Autodesk Inventor part; units mm, degrees
(part 2 of 4)
sketch "Sketch5" plane through (0, 0, 0) normal (-1, 0, 0) x (0, 0, 1)
  line L0 (0, 0) -> (304.8, 0) projected
  line L1 (0, 0) -> (0, -25.4) projected
  line L2 (304.8, -25.4) -> (0, -25.4) projected
  line L3 (304.8, 0) -> (304.8, -25.4) projected
  line L4 (24.765, -3.175) -> (24.765, -22.225)
  line L5 (24.765, -22.225) -> (26.035, -22.225)
  line L6 (26.035, -22.225) -> (26.035, -3.175)
  line L7 (26.035, -3.175) -> (24.765, -3.175)
  line L8 (6.0325, -6.35) -> (18.7325, -6.35) construction
  line L9 (18.7325, -6.35) -> (18.7325, -19.05) construction
  line L10 (18.7325, -19.05) -> (6.0325, -19.05) construction
  line L11 (6.0325, -19.05) -> (6.0325, -6.35) construction
  line L12 (50.165, -3.175) -> (50.165, -22.225)
  line L13 (51.435, -3.175) -> (50.165, -3.175)
  line L14 (50.165, -22.225) -> (51.435, -22.225)
  line L15 (51.435, -22.225) -> (51.435, -3.175)
  line L16 (75.565, -3.175) -> (75.565, -22.225)
  line L17 (76.835, -3.175) -> (75.565, -3.175)
  line L18 (75.565, -22.225) -> (76.835, -22.225)
  line L19 (76.835, -22.225) -> (76.835, -3.175)
  line L20 (100.965, -3.175) -> (100.965, -22.225)
  line L21 (102.235, -3.175) -> (100.965, -3.175)
  line L22 (100.965, -22.225) -> (102.235, -22.225)
  line L23 (102.235, -22.225) -> (102.235, -3.175)
  line L24 (126.365, -3.175) -> (126.365, -22.225)
  line L25 (127.635, -3.175) -> (126.365, -3.175)
  line L26 (126.365, -22.225) -> (127.635, -22.225)
  line L27 (127.635, -22.225) -> (127.635, -3.175)
  line L28 (151.765, -3.175) -> (151.765, -22.225)
  line L29 (153.035, -3.175) -> (151.765, -3.175)
  line L30 (151.765, -22.225) -> (153.035, -22.225)
  line L31 (153.035, -22.225) -> (153.035, -3.175)
  line L32 (177.165, -3.175) -> (177.165, -22.225)
  line L33 (178.435, -3.175) -> (177.165, -3.175)
  line L34 (177.165, -22.225) -> (178.435, -22.225)
  line L35 (178.435, -22.225) -> (178.435, -3.175)
  line L36 (202.565, -3.175) -> (202.565, -22.225)
  line L37 (203.835, -3.175) -> (202.565, -3.175)
  line L38 (202.565, -22.225) -> (203.835, -22.225)
  line L39 (203.835, -22.225) -> (203.835, -3.175)
  line L40 (227.965, -3.175) -> (227.965, -22.225)
  line L41 (229.235, -3.175) -> (227.965, -3.175)
  line L42 (227.965, -22.225) -> (229.235, -22.225)
  line L43 (229.235, -22.225) -> (229.235, -3.175)
  line L44 (253.365, -3.175) -> (253.365, -22.225)
  line L45 (254.635, -3.175) -> (253.365, -3.175)
  line L46 (253.365, -22.225) -> (254.635, -22.225)
  line L47 (254.635, -22.225) -> (254.635, -3.175)
  line L48 (278.765, -3.175) -> (278.765, -22.225)
  line L49 (280.035, -3.175) -> (278.765, -3.175)
  line L50 (278.765, -22.225) -> (280.035, -22.225)
  line L51 (280.035, -22.225) -> (280.035, -3.175)
  line L52 (31.4325, -6.35) -> (44.1325, -6.35) construction
  line L53 (44.1325, -6.35) -> (44.1325, -19.05) construction
  line L54 (44.1325, -19.05) -> (31.4325, -19.05) construction
  line L55 (31.4325, -19.05) -> (31.4325, -6.35) construction
  line L56 (56.8325, -6.35) -> (69.5325, -6.35) construction
  line L57 (69.5325, -6.35) -> (69.5325, -19.05) construction
  line L58 (69.5325, -19.05) -> (56.8325, -19.05) construction
  line L59 (56.8325, -19.05) -> (56.8325, -6.35) construction
  line L60 (82.2325, -6.35) -> (94.9325, -6.35) construction
  line L61 (94.9325, -6.35) -> (94.9325, -19.05) construction
  line L62 (94.9325, -19.05) -> (82.2325, -19.05) construction
  line L63 (82.2325, -19.05) -> (82.2325, -6.35) construction
  line L64 (107.6325, -6.35) -> (120.3325, -6.35) construction
  line L65 (120.3325, -6.35) -> (120.3325, -19.05) construction
  line L66 (120.3325, -19.05) -> (107.6325, -19.05) construction
  line L67 (107.6325, -19.05) -> (107.6325, -6.35) construction
  line L68 (133.0325, -6.35) -> (145.7325, -6.35) construction
  line L69 (145.7325, -6.35) -> (145.7325, -19.05) construction
  line L70 (145.7325, -19.05) -> (133.0325, -19.05) construction
  line L71 (133.0325, -19.05) -> (133.0325, -6.35) construction
  line L72 (158.4325, -6.35) -> (171.1325, -6.35) construction
  line L73 (171.1325, -6.35) -> (171.1325, -19.05) construction
  line L74 (171.1325, -19.05) -> (158.4325, -19.05) construction
  line L75 (158.4325, -19.05) -> (158.4325, -6.35) construction
  line L76 (183.8325, -6.35) -> (196.5325, -6.35) construction
  line L77 (196.5325, -6.35) -> (196.5325, -19.05) construction
  line L78 (196.5325, -19.05) -> (183.8325, -19.05) construction
  line L79 (183.8325, -19.05) -> (183.8325, -6.35) construction
  line L80 (209.2325, -6.35) -> (221.9325, -6.35) construction
  line L81 (221.9325, -6.35) -> (221.9325, -19.05) construction
  line L82 (221.9325, -19.05) -> (209.2325, -19.05) construction
  line L83 (209.2325, -19.05) -> (209.2325, -6.35) construction
  line L84 (234.6325, -6.35) -> (247.3325, -6.35) construction
  line L85 (247.3325, -6.35) -> (247.3325, -19.05) construction
  line L86 (247.3325, -19.05) -> (234.6325, -19.05) construction
  line L87 (234.6325, -19.05) -> (234.6325, -6.35) construction
  line L88 (260.0325, -6.35) -> (272.7325, -6.35) construction
  line L89 (272.7325, -6.35) -> (272.7325, -19.05) construction
  line L90 (272.7325, -19.05) -> (260.0325, -19.05) construction
  line L91 (260.0325, -19.05) -> (260.0325, -6.35) construction
  line L92 (285.4325, -6.35) -> (298.1325, -6.35) construction
  line L93 (298.1325, -6.35) -> (298.1325, -19.05) construction
  line L94 (298.1325, -19.05) -> (285.4325, -19.05) construction
  line L95 (285.4325, -19.05) -> (285.4325, -6.35) construction
  line L96 (29.3758, -17.272) -> (32.4584, -8.128)
  line L97 (32.4584, -8.128) -> (33.9552, -8.128)
  line L98 (33.9552, -8.128) -> (37.0378, -17.272)
  line L99 (37.0378, -17.272) -> (35.7559, -17.272)
  line L100 (35.7559, -17.272) -> (34.9259, -14.7155)
  line L101 (34.9259, -14.7155) -> (31.4358, -14.7155)
  line L102 (31.4358, -14.7155) -> (30.6059, -17.272)
  line L103 (30.6059, -17.272) -> (29.3758, -17.272)
  line L104 (34.5925, -13.6781) -> (33.1772, -9.3729)
  line L105 (33.1772, -9.3729) -> (31.7692, -13.6781)
  line L106 (31.7692, -13.6781) -> (34.5925, -13.6781)
  line L107 (45.2629, -11.5514) -> (43.4623, -11.5514)
  line L108 (43.4623, -11.5514) -> (42.9065, -13.856)
  line L109 (42.9065, -13.856) -> (44.5442, -13.856)
  line L110 (44.5442, -13.856) -> (44.5442, -14.6859)
  line L111 (44.5442, -14.6859) -> (42.6917, -14.6859)
  line L112 (42.6917, -14.6859) -> (42.047, -17.272)
  line L113 (42.047, -17.272) -> (41.2541, -17.272)
  line L114 (41.2541, -17.272) -> (41.8988, -14.6859)
  line L115 (41.8988, -14.6859) -> (40.2241, -14.6859)
  line L116 (40.2241, -14.6859) -> (39.5794, -17.272)
  line L117 (39.5794, -17.272) -> (38.7866, -17.272)
  line L118 (38.7866, -17.272) -> (39.4312, -14.6859)
  line L119 (39.4312, -14.6859) -> (37.8455, -14.6859)
  line L120 (37.8455, -14.6859) -> (37.8455, -13.856)
  line L121 (37.8455, -13.856) -> (39.6461, -13.856)
  line L122 (39.6461, -13.856) -> (40.2019, -11.5514)
  line L123 (40.2019, -11.5514) -> (38.5643, -11.5514)
  line L124 (38.5643, -11.5514) -> (38.5643, -10.7215)
  line L125 (38.5643, -10.7215) -> (40.4168, -10.7215)
  line L126 (40.4168, -10.7215) -> (41.0614, -8.128)
  line L127 (41.0614, -8.128) -> (41.8543, -8.128)
  line L128 (41.8543, -8.128) -> (41.2096, -10.7215)
  line L129 (41.2096, -10.7215) -> (42.8843, -10.7215)
  line L130 (42.8843, -10.7215) -> (43.529, -8.128)
  line L131 (43.529, -8.128) -> (44.3219, -8.128)
  line L132 (44.3219, -8.128) -> (43.6772, -10.7215)
  line L133 (43.6772, -10.7215) -> (45.2629, -10.7215)
  line L134 (45.2629, -10.7215) -> (45.2629, -11.5514)
  line L135 (42.6917, -11.5366) -> (40.9948, -11.5366)
  line L136 (40.9948, -11.5366) -> (40.4242, -13.8708)
  line L137 (40.4242, -13.8708) -> (42.1211, -13.8708)
  line L138 (42.1211, -13.8708) -> (42.6917, -11.5366)
  spline S0 degree 2 poles (15.8059, -14.4636) (15.8059, -15.1453) (15.2872, -16.1901) (14.8575, -16.531) knots 0 0 0 1 2 2 2
  spline S1 degree 2 poles (14.8575, -16.531) (14.3388, -16.9311) (13.1606, -17.272) (12.2269, -17.272) knots 0 0 0 1 2 2 2
  line L139 (12.2269, -17.272) -> (9.6037, -17.272)
  line L140 (9.6037, -17.272) -> (9.6037, -8.128)
  line L141 (9.6037, -8.128) -> (12.0268, -8.128)
  spline S2 degree 2 poles (12.0268, -8.128) (13.0049, -8.128) (13.9831, -8.254) (14.4277, -8.4985) knots 0 0 0 1 2 2 2
  spline S3 degree 2 poles (14.4277, -8.4985) (14.9241, -8.7579) (15.3762, -9.61) (15.3762, -10.188) knots 0 0 0 1 2 2 2
  spline S4 degree 2 poles (15.3762, -10.188) (15.3762, -10.8327) (14.6944, -11.8553) (14.0942, -12.1442) knots 0 0 0 1 2 2 2
  line L142 (14.0942, -12.1442) -> (14.0942, -12.1887)
  spline S5 degree 2 poles (14.0942, -12.1887) (14.9093, -12.411) (15.8059, -13.5892) (15.8059, -14.4636) knots 0 0 0 1 2 2 2
  spline S6 degree 2 poles (14.5388, -14.5155) (14.5388, -13.9968) (14.2424, -13.3299) (13.7978, -13.0927) knots 0 0 0 1 2 2 2
  spline S7 degree 2 poles (13.7978, -13.0927) (13.5088, -12.9445) (12.8271, -12.8556) (12.1972, -12.8556) knots 0 0 0 1 2 2 2
  line L143 (12.1972, -12.8556) -> (10.819, -12.8556)
  line L144 (10.819, -12.8556) -> (10.819, -16.2346)
  line L145 (10.819, -16.2346) -> (11.8045, -16.2346)
  spline S8 degree 2 poles (11.8045, -16.2346) (12.6048, -16.2346) (13.5236, -16.0864) (13.8793, -15.8493) knots 0 0 0 1 2 2 2
  spline S9 degree 2 poles (13.8793, -15.8493) (14.2202, -15.6047) (14.5388, -14.9971) (14.5388, -14.5155) knots 0 0 0 1 2 2 2
  spline S10 degree 2 poles (14.109, -10.3584) (14.109, -10.0324) (13.8867, -9.5433) (13.6422, -9.4025) knots 0 0 0 1 2 2 2
  spline S11 degree 2 poles (13.6422, -9.4025) (13.3458, -9.2395) (12.627, -9.1654) (11.9824, -9.1654) knots 0 0 0 1 2 2 2
  line L146 (11.9824, -9.1654) -> (10.819, -9.1654)
  line L147 (10.819, -9.1654) -> (10.819, -11.8404)
  line L148 (10.819, -11.8404) -> (12.1972, -11.8404)
  spline S12 degree 2 poles (12.1972, -11.8404) (12.7678, -11.8404) (13.3088, -11.7219) (13.5977, -11.5366) knots 0 0 0 1 2 2 2
  spline S13 degree 2 poles (13.5977, -11.5366) (13.8793, -11.3588) (14.109, -10.7882) (14.109, -10.3584) knots 0 0 0 1 2 2 2
  line L149 (59.2922, -17.272) -> (62.3748, -8.128)
  line L150 (62.3748, -8.128) -> (63.8716, -8.128)
  line L151 (63.8716, -8.128) -> (66.9542, -17.272)
  line L152 (66.9542, -17.272) -> (65.6723, -17.272)
  line L153 (65.6723, -17.272) -> (64.8424, -14.7155)
  line L154 (64.8424, -14.7155) -> (61.3522, -14.7155)
  line L155 (61.3522, -14.7155) -> (60.5223, -17.272)
  line L156 (60.5223, -17.272) -> (59.2922, -17.272)
  line L157 (64.5089, -13.6781) -> (63.0936, -9.3729)
  line L158 (63.0936, -9.3729) -> (61.6857, -13.6781)
  line L159 (61.6857, -13.6781) -> (64.5089, -13.6781)
  spline S14 degree 2 poles (84.5663, -17.4424) (83.5955, -17.4424) (81.9876, -16.8496) (81.4096, -16.2494) knots 0 0 0 1 2 2 2
  spline S15 degree 2 poles (81.4096, -16.2494) (80.8316, -15.6418) (80.2166, -13.8486) (80.2166, -12.6852) knots 0 0 0 1 2 2 2
  spline S16 degree 2 poles (80.2166, -12.6852) (80.2166, -11.5811) (80.839, -9.8323) (81.417, -9.2099) knots 0 0 0 1 2 2 2
  spline S17 degree 2 poles (81.417, -9.2099) (81.9727, -8.6097) (83.6029, -7.9576) (84.5737, -7.9576) knots 0 0 0 1 2 2 2
  spline S18 degree 2 poles (84.5737, -7.9576) (85.0405, -7.9576) (85.8852, -8.0909) (86.2706, -8.2095) knots 0 0 0 1 2 2 2
  spline S19 degree 2 poles (86.2706, -8.2095) (86.5818, -8.2984) (87.3376, -8.6245) (87.5673, -8.743) knots 0 0 0 1 2 2 2
  line L160 (87.5673, -8.743) -> (87.5673, -10.2102)
  line L161 (87.5673, -10.2102) -> (87.4636, -10.2102)
  spline S20 degree 2 poles (87.4636, -10.2102) (87.2339, -10.0102) (86.7522, -9.6471) (86.3076, -9.4396) knots 0 0 0 1 2 2 2
  spline S21 degree 2 poles (86.3076, -9.4396) (85.9371, -9.2543) (84.9812, -9.0098) (84.4329, -9.0098) knots 0 0 0 1 2 2 2
  spline S22 degree 2 poles (84.4329, -9.0098) (83.1139, -9.0098) (81.4837, -10.9957) (81.4837, -12.6481) knots 0 0 0 1 2 2 2
  spline S23 degree 2 poles (81.4837, -12.6481) (81.4837, -13.567) (81.9135, -14.9452) (82.321, -15.4195) knots 0 0 0 1 2 2 2
  spline S24 degree 2 poles (82.321, -15.4195) (82.7137, -15.8937) (83.8252, -16.3902) (84.5218, -16.3902) knots 0 0 0 1 2 2 2
  spline S25 degree 2 poles (84.5218, -16.3902) (85.0331, -16.3902) (86.0557, -16.242) (86.4039, -16.0938) knots 0 0 0 1 2 2 2
  line L162 (86.4039, -16.0938) -> (86.4039, -13.73)
  line L163 (86.4039, -13.73) -> (84.2847, -13.73)
  line L164 (84.2847, -13.73) -> (84.2847, -12.6629)
  line L165 (84.2847, -12.6629) -> (87.6044, -12.6629)
  line L166 (87.6044, -12.6629) -> (87.6044, -16.657)
  spline S26 degree 2 poles (87.6044, -16.657) (87.3747, -16.7607) (86.5892, -17.0793) (86.2557, -17.1757) knots 0 0 0 1 2 2 2
  spline S27 degree 2 poles (86.2557, -17.1757) (85.8037, -17.3091) (85.0775, -17.4424) (84.5663, -17.4424) knots 0 0 0 1 2 2 2
  line L167 (96.489, -11.544) -> (94.6884, -11.544)
  line L168 (94.6884, -11.544) -> (94.1326, -13.8486)
  line L169 (94.1326, -13.8486) -> (95.7702, -13.8486)
  line L170 (95.7702, -13.8486) -> (95.7702, -14.6785)
  line L171 (95.7702, -14.6785) -> (93.9177, -14.6785)
  line L172 (93.9177, -14.6785) -> (93.2731, -17.2646)
  line L173 (93.2731, -17.2646) -> (92.4802, -17.2646)
  line L174 (92.4802, -17.2646) -> (93.1249, -14.6785)
  line L175 (93.1249, -14.6785) -> (91.4502, -14.6785)
  line L176 (91.4502, -14.6785) -> (90.8055, -17.2646)
  line L177 (90.8055, -17.2646) -> (90.0126, -17.2646)
  line L178 (90.0126, -17.2646) -> (90.6573, -14.6785)
  line L179 (90.6573, -14.6785) -> (89.0716, -14.6785)
  line L180 (89.0716, -14.6785) -> (89.0716, -13.8486)
  line L181 (89.0716, -13.8486) -> (90.8722, -13.8486)
  line L182 (90.8722, -13.8486) -> (91.428, -11.544)
  line L183 (91.428, -11.544) -> (89.7903, -11.544)
  line L184 (89.7903, -11.544) -> (89.7903, -10.7141)
  line L185 (89.7903, -10.7141) -> (91.6428, -10.7141)
  line L186 (91.6428, -10.7141) -> (92.2875, -8.1206)
  line L187 (92.2875, -8.1206) -> (93.0804, -8.1206)
  line L188 (93.0804, -8.1206) -> (92.4357, -10.7141)
  line L189 (92.4357, -10.7141) -> (94.1104, -10.7141)
  line L190 (94.1104, -10.7141) -> (94.7551, -8.1206)
  line L191 (94.7551, -8.1206) -> (95.5479, -8.1206)
  line L192 (95.5479, -8.1206) -> (94.9033, -10.7141)
  line L193 (94.9033, -10.7141) -> (96.489, -10.7141)
  line L194 (96.489, -10.7141) -> (96.489, -11.544)
  line L195 (93.9177, -11.5292) -> (92.2208, -11.5292)
  line L196 (92.2208, -11.5292) -> (91.6503, -13.8634)
  line L197 (91.6503, -13.8634) -> (93.3472, -13.8634)
  line L198 (93.3472, -13.8634) -> (93.9177, -11.5292)
  spline S28 degree 2 poles (114.542, -17.4424) (113.5712, -17.4424) (111.9633, -16.8496) (111.3853, -16.2494) knots 0 0 0 1 2 2 2
  spline S29 degree 2 poles (111.3853, -16.2494) (110.8073, -15.6418) (110.1923, -13.8486) (110.1923, -12.6852) knots 0 0 0 1 2 2 2
  spline S30 degree 2 poles (110.1923, -12.6852) (110.1923, -11.5811) (110.8147, -9.8323) (111.3927, -9.2099) knots 0 0 0 1 2 2 2
  spline S31 degree 2 poles (111.3927, -9.2099) (111.9484, -8.6097) (113.5787, -7.9576) (114.5494, -7.9576) knots 0 0 0 1 2 2 2
  spline S32 degree 2 poles (114.5494, -7.9576) (115.0162, -7.9576) (115.8609, -8.0909) (116.2463, -8.2095) knots 0 0 0 1 2 2 2
  spline S33 degree 2 poles (116.2463, -8.2095) (116.5575, -8.2984) (117.3133, -8.6245) (117.543, -8.743) knots 0 0 0 1 2 2 2
  line L199 (117.543, -8.743) -> (117.543, -10.2102)
  line L200 (117.543, -10.2102) -> (117.4393, -10.2102)
  spline S34 degree 2 poles (117.4393, -10.2102) (117.2096, -10.0102) (116.7279, -9.6471) (116.2833, -9.4396) knots 0 0 0 1 2 2 2
  spline S35 degree 2 poles (116.2833, -9.4396) (115.9128, -9.2543) (114.9569, -9.0098) (114.4086, -9.0098) knots 0 0 0 1 2 2 2
  spline S36 degree 2 poles (114.4086, -9.0098) (113.0896, -9.0098) (111.4594, -10.9957) (111.4594, -12.6481) knots 0 0 0 1 2 2 2
  spline S37 degree 2 poles (111.4594, -12.6481) (111.4594, -13.567) (111.8892, -14.9452) (112.2967, -15.4195) knots 0 0 0 1 2 2 2
  spline S38 degree 2 poles (112.2967, -15.4195) (112.6894, -15.8937) (113.801, -16.3902) (114.4975, -16.3902) knots 0 0 0 1 2 2 2
  spline S39 degree 2 poles (114.4975, -16.3902) (115.0088, -16.3902) (116.0314, -16.242) (116.3796, -16.0938) knots 0 0 0 1 2 2 2
  line L201 (116.3796, -16.0938) -> (116.3796, -13.73)
  line L202 (116.3796, -13.73) -> (114.2604, -13.73)
  line L203 (114.2604, -13.73) -> (114.2604, -12.6629)
  line L204 (114.2604, -12.6629) -> (117.5801, -12.6629)
  line L205 (117.5801, -12.6629) -> (117.5801, -16.657)
  spline S40 degree 2 poles (117.5801, -16.657) (117.3504, -16.7607) (116.5649, -17.0793) (116.2314, -17.1757) knots 0 0 0 1 2 2 2
  spline S41 degree 2 poles (116.2314, -17.1757) (115.7794, -17.3091) (115.0533, -17.4424) (114.542, -17.4424) knots 0 0 0 1 2 2 2
  line L206 (137.9227, -9.2099) -> (133.6694, -9.2099)
  line L207 (133.6694, -9.2099) -> (133.6694, -11.7886)
  line L208 (133.6694, -11.7886) -> (137.7449, -11.7886)
  line L209 (137.7449, -11.7886) -> (137.7449, -12.8704)
  line L210 (137.7449, -12.8704) -> (133.6694, -12.8704)
  line L211 (133.6694, -12.8704) -> (133.6694, -17.272)
  line L212 (133.6694, -17.272) -> (132.4541, -17.272)
  line L213 (132.4541, -17.272) -> (132.4541, -8.128)
  line L214 (132.4541, -8.128) -> (137.9227, -8.128)
  line L215 (137.9227, -8.128) -> (137.9227, -9.2099)
  line L216 (146.3702, -11.5514) -> (144.5695, -11.5514)
  line L217 (144.5695, -11.5514) -> (144.0138, -13.856)
  line L218 (144.0138, -13.856) -> (145.6514, -13.856)
  line L219 (145.6514, -13.856) -> (145.6514, -14.6859)
  line L220 (145.6514, -14.6859) -> (143.7989, -14.6859)
  line L221 (143.7989, -14.6859) -> (143.1542, -17.272)
  line L222 (143.1542, -17.272) -> (142.3613, -17.272)
  line L223 (142.3613, -17.272) -> (143.006, -14.6859)
  line L224 (143.006, -14.6859) -> (141.3313, -14.6859)
  line L225 (141.3313, -14.6859) -> (140.6867, -17.272)
  line L226 (140.6867, -17.272) -> (139.8938, -17.272)
  line L227 (139.8938, -17.272) -> (140.5385, -14.6859)
  line L228 (140.5385, -14.6859) -> (138.9527, -14.6859)
  line L229 (138.9527, -14.6859) -> (138.9527, -13.856)
  line L230 (138.9527, -13.856) -> (140.7534, -13.856)
  line L231 (140.7534, -13.856) -> (141.3091, -11.5514)
  line L232 (141.3091, -11.5514) -> (139.6715, -11.5514)
  line L233 (139.6715, -11.5514) -> (139.6715, -10.7215)
  line L234 (139.6715, -10.7215) -> (141.524, -10.7215)
  line L235 (141.524, -10.7215) -> (142.1687, -8.128)
  line L236 (142.1687, -8.128) -> (142.9616, -8.128)
  line L237 (142.9616, -8.128) -> (142.3169, -10.7215)
  line L238 (142.3169, -10.7215) -> (143.9915, -10.7215)
  line L239 (143.9915, -10.7215) -> (144.6362, -8.128)
  line L240 (144.6362, -8.128) -> (145.4291, -8.128)
  line L241 (145.4291, -8.128) -> (144.7844, -10.7215)
  line L242 (144.7844, -10.7215) -> (146.3702, -10.7215)
  line L243 (146.3702, -10.7215) -> (146.3702, -11.5514)
  line L244 (143.7989, -11.5366) -> (142.102, -11.5366)
  line L245 (142.102, -11.5366) -> (141.5314, -13.8708)
  line L246 (141.5314, -13.8708) -> (143.2283, -13.8708)
  line L247 (143.2283, -13.8708) -> (143.7989, -11.5366)
  line L248 (167.8984, -9.2099) -> (163.6451, -9.2099)
  line L249 (163.6451, -9.2099) -> (163.6451, -11.7886)
  line L250 (163.6451, -11.7886) -> (167.7206, -11.7886)
  line L251 (167.7206, -11.7886) -> (167.7206, -12.8704)
  line L252 (167.7206, -12.8704) -> (163.6451, -12.8704)
  line L253 (163.6451, -12.8704) -> (163.6451, -17.272)
  line L254 (163.6451, -17.272) -> (162.4298, -17.272)
  line L255 (162.4298, -17.272) -> (162.4298, -8.128)
  line L256 (162.4298, -8.128) -> (167.8984, -8.128)
  line L257 (167.8984, -8.128) -> (167.8984, -9.2099)
  line L258 (187.5816, -17.272) -> (187.5816, -8.128)
  line L259 (187.5816, -8.128) -> (193.3021, -8.128)
  line L260 (193.3021, -8.128) -> (193.3021, -9.2099)
  line L261 (193.3021, -9.2099) -> (188.7968, -9.2099)
  line L262 (188.7968, -9.2099) -> (188.7968, -11.7145)
  line L263 (188.7968, -11.7145) -> (192.9983, -11.7145)
  line L264 (192.9983, -11.7145) -> (192.9983, -12.7963)
  line L265 (192.9983, -12.7963) -> (188.7968, -12.7963)
  line L266 (188.7968, -12.7963) -> (188.7968, -16.1901)
  line L267 (188.7968, -16.1901) -> (193.3021, -16.1901)
  line L268 (193.3021, -16.1901) -> (193.3021, -17.272)
  line L269 (193.3021, -17.272) -> (187.5816, -17.272)
  spline S42 degree 2 poles (214.8785, -12.7074) (214.8785, -13.9597) (213.8634, -15.9752) (213.0112, -16.5384) knots 0 0 0 1 2 2 2
  spline S43 degree 2 poles (213.0112, -16.5384) (212.3147, -16.9756) (210.8845, -17.272) (209.773, -17.272) knots 0 0 0 1 2 2 2
  line L270 (209.773, -17.272) -> (207.6686, -17.272)
  line L271 (207.6686, -17.272) -> (207.6686, -8.128)
  line L272 (207.6686, -8.128) -> (209.7508, -8.128)
  spline S44 degree 2 poles (209.7508, -8.128) (211.0401, -8.128) (212.5073, -8.5133) (213.026, -8.8542) knots 0 0 0 1 2 2 2
  spline S45 degree 2 poles (213.026, -8.8542) (213.9078, -9.4396) (214.8785, -11.3736) (214.8785, -12.7074) knots 0 0 0 1 2 2 2
  spline S46 degree 2 poles (213.6114, -12.6926) (213.6114, -11.6404) (212.9149, -10.1509) (212.2257, -9.7286) knots 0 0 0 1 2 2 2
  spline S47 degree 2 poles (212.2257, -9.7286) (211.7367, -9.4396) (210.6326, -9.1802) (209.8101, -9.1802) knots 0 0 0 1 2 2 2
  line L273 (209.8101, -9.1802) -> (208.8838, -9.1802)
  line L274 (208.8838, -9.1802) -> (208.8838, -16.2198)
  line L275 (208.8838, -16.2198) -> (209.8101, -16.2198)
  spline S48 degree 2 poles (209.8101, -16.2198) (210.6178, -16.2198) (211.8404, -15.9604) (212.3369, -15.6121) knots 0 0 0 1 2 2 2
  spline S49 degree 2 poles (212.3369, -15.6121) (212.9742, -15.1824) (213.6114, -13.7596) (213.6114, -12.6926) knots 0 0 0 1 2 2 2
  line L276 (223.5557, -11.5514) -> (221.7551, -11.5514)
  line L277 (221.7551, -11.5514) -> (221.1993, -13.856)
  line L278 (221.1993, -13.856) -> (222.8369, -13.856)
  line L279 (222.8369, -13.856) -> (222.8369, -14.6859)
  line L280 (222.8369, -14.6859) -> (220.9844, -14.6859)
  line L281 (220.9844, -14.6859) -> (220.3397, -17.272)
  line L282 (220.3397, -17.272) -> (219.5469, -17.272)
  line L283 (219.5469, -17.272) -> (220.1915, -14.6859)
  line L284 (220.1915, -14.6859) -> (218.5169, -14.6859)
  line L285 (218.5169, -14.6859) -> (217.8722, -17.272)
  line L286 (217.8722, -17.272) -> (217.0793, -17.272)
  line L287 (217.0793, -17.272) -> (217.724, -14.6859)
  line L288 (217.724, -14.6859) -> (216.1383, -14.6859)
  line L289 (216.1383, -14.6859) -> (216.1383, -13.856)
  line L290 (216.1383, -13.856) -> (217.9389, -13.856)
  line L291 (217.9389, -13.856) -> (218.4946, -11.5514)
  line L292 (218.4946, -11.5514) -> (216.857, -11.5514)
  line L293 (216.857, -11.5514) -> (216.857, -10.7215)
  line L294 (216.857, -10.7215) -> (218.7095, -10.7215)
  line L295 (218.7095, -10.7215) -> (219.3542, -8.128)
  line L296 (219.3542, -8.128) -> (220.1471, -8.128)
  line L297 (220.1471, -8.128) -> (219.5024, -10.7215)
  line L298 (219.5024, -10.7215) -> (221.1771, -10.7215)
  line L299 (221.1771, -10.7215) -> (221.8218, -8.128)
  line L300 (221.8218, -8.128) -> (222.6146, -8.128)
  line L301 (222.6146, -8.128) -> (221.97, -10.7215)
  line L302 (221.97, -10.7215) -> (223.5557, -10.7215)
  line L303 (223.5557, -10.7215) -> (223.5557, -11.5514)
  line L304 (220.9844, -11.5366) -> (219.2875, -11.5366)
  line L305 (219.2875, -11.5366) -> (218.7169, -13.8708)
  line L306 (218.7169, -13.8708) -> (220.4138, -13.8708)
  line L307 (220.4138, -13.8708) -> (220.9844, -11.5366)
  spline S50 degree 2 poles (244.8542, -12.7074) (244.8542, -13.9597) (243.8391, -15.9752) (242.9869, -16.5384) knots 0 0 0 1 2 2 2
  spline S51 degree 2 poles (242.9869, -16.5384) (242.2904, -16.9756) (240.8602, -17.272) (239.7487, -17.272) knots 0 0 0 1 2 2 2
  line L308 (239.7487, -17.272) -> (237.6443, -17.272)
  line L309 (237.6443, -17.272) -> (237.6443, -8.128)
  line L310 (237.6443, -8.128) -> (239.7265, -8.128)
  spline S52 degree 2 poles (239.7265, -8.128) (241.0158, -8.128) (242.483, -8.5133) (243.0017, -8.8542) knots 0 0 0 1 2 2 2
  spline S53 degree 2 poles (243.0017, -8.8542) (243.8835, -9.4396) (244.8542, -11.3736) (244.8542, -12.7074) knots 0 0 0 1 2 2 2
  spline S54 degree 2 poles (243.5871, -12.6926) (243.5871, -11.6404) (242.8906, -10.1509) (242.2014, -9.7286) knots 0 0 0 1 2 2 2
  spline S55 degree 2 poles (242.2014, -9.7286) (241.7124, -9.4396) (240.6083, -9.1802) (239.7858, -9.1802) knots 0 0 0 1 2 2 2
  line L311 (239.7858, -9.1802) -> (238.8595, -9.1802)
  line L312 (238.8595, -9.1802) -> (238.8595, -16.2198)
  line L313 (238.8595, -16.2198) -> (239.7858, -16.2198)
  spline S56 degree 2 poles (239.7858, -16.2198) (240.5935, -16.2198) (241.8161, -15.9604) (242.3126, -15.6121) knots 0 0 0 1 2 2 2
  spline S57 degree 2 poles (242.3126, -15.6121) (242.9499, -15.1824) (243.5871, -13.7596) (243.5871, -12.6926) knots 0 0 0 1 2 2 2
  spline S58 degree 2 poles (262.5293, -17.435) (261.6401, -17.435) (260.1358, -16.8348) (259.5875, -16.2346) knots 0 0 0 1 2 2 2
  spline S59 degree 2 poles (259.5875, -16.2346) (259.0391, -15.6418) (258.4389, -13.8634) (258.4389, -12.7074) knots 0 0 0 1 2 2 2
  spline S60 degree 2 poles (258.4389, -12.7074) (258.4389, -11.5589) (259.0243, -9.8545) (259.5801, -9.2247) knots 0 0 0 1 2 2 2
  spline S61 degree 2 poles (259.5801, -9.2247) (260.1284, -8.6097) (261.6252, -7.965) (262.5515, -7.965) knots 0 0 0 1 2 2 2
  spline S62 degree 2 poles (262.5515, -7.965) (263.0109, -7.965) (263.8186, -8.0984) (264.1595, -8.2021) knots 0 0 0 1 2 2 2
  spline S63 degree 2 poles (264.1595, -8.2021) (264.4559, -8.2984) (265.0709, -8.5726) (265.3747, -8.7356) knots 0 0 0 1 2 2 2
  line L314 (265.3747, -8.7356) -> (265.3747, -10.2028)
  line L315 (265.3747, -10.2028) -> (265.2784, -10.2028)
  spline S64 degree 2 poles (265.2784, -10.2028) (265.1154, -10.0546) (264.6115, -9.6396) (264.2484, -9.4396) knots 0 0 0 1 2 2 2
  spline S65 degree 2 poles (264.2484, -9.4396) (263.9001, -9.2469) (263.0776, -9.0024) (262.5441, -9.0024) knots 0 0 0 1 2 2 2
  spline S66 degree 2 poles (262.5441, -9.0024) (261.9587, -9.0024) (260.9139, -9.484) (260.5211, -9.9435) knots 0 0 0 1 2 2 2
  spline S67 degree 2 poles (260.5211, -9.9435) (260.1358, -10.4103) (259.706, -11.8256) (259.706, -12.7074) knots 0 0 0 1 2 2 2
  spline S68 degree 2 poles (259.706, -12.7074) (259.706, -13.6485) (260.1581, -15.0045) (260.5508, -15.4714) knots 0 0 0 1 2 2 2
  spline S69 degree 2 poles (260.5508, -15.4714) (260.9361, -15.9234) (261.9661, -16.3828) (262.5441, -16.3828) knots 0 0 0 1 2 2 2
  spline S70 degree 2 poles (262.5441, -16.3828) (263.0702, -16.3828) (263.9668, -16.1234) (264.3151, -15.9308) knots 0 0 0 1 2 2 2
  spline S71 degree 2 poles (264.3151, -15.9308) (264.6485, -15.7381) (265.145, -15.338) (265.2858, -15.1972) knots 0 0 0 1 2 2 2
  line L316 (265.2858, -15.1972) -> (265.3747, -15.1972)
  line L317 (265.3747, -15.1972) -> (265.3747, -16.6496)
  spline S72 degree 2 poles (265.3747, -16.6496) (265.0709, -16.7903) (264.5374, -17.0497) (264.1595, -17.1683) knots 0 0 0 1 2 2 2
  spline S73 degree 2 poles (264.1595, -17.1683) (263.7593, -17.3016) (263.0776, -17.435) (262.5293, -17.435) knots 0 0 0 1 2 2 2
  line L318 (273.8666, -11.5514) -> (272.066, -11.5514)
  line L319 (272.066, -11.5514) -> (271.5102, -13.856)
  line L320 (271.5102, -13.856) -> (273.1479, -13.856)
  line L321 (273.1479, -13.856) -> (273.1479, -14.6859)
  line L322 (273.1479, -14.6859) -> (271.2954, -14.6859)
  line L323 (271.2954, -14.6859) -> (270.6507, -17.272)
  line L324 (270.6507, -17.272) -> (269.8578, -17.272)
  line L325 (269.8578, -17.272) -> (270.5025, -14.6859)
  line L326 (270.5025, -14.6859) -> (268.8278, -14.6859)
  line L327 (268.8278, -14.6859) -> (268.1831, -17.272)
  line L328 (268.1831, -17.272) -> (267.3903, -17.272)
  line L329 (267.3903, -17.272) -> (268.0349, -14.6859)
  line L330 (268.0349, -14.6859) -> (266.4492, -14.6859)
  line L331 (266.4492, -14.6859) -> (266.4492, -13.856)
  line L332 (266.4492, -13.856) -> (268.2498, -13.856)
  line L333 (268.2498, -13.856) -> (268.8056, -11.5514)
  line L334 (268.8056, -11.5514) -> (267.168, -11.5514)
  line L335 (267.168, -11.5514) -> (267.168, -10.7215)
  line L336 (267.168, -10.7215) -> (269.0205, -10.7215)
  line L337 (269.0205, -10.7215) -> (269.6651, -8.128)
  line L338 (269.6651, -8.128) -> (270.458, -8.128)
  line L339 (270.458, -8.128) -> (269.8133, -10.7215)
  line L340 (269.8133, -10.7215) -> (271.488, -10.7215)
  line L341 (271.488, -10.7215) -> (272.1327, -8.128)
  line L342 (272.1327, -8.128) -> (272.9256, -8.128)
  line L343 (272.9256, -8.128) -> (272.2809, -10.7215)
  line L344 (272.2809, -10.7215) -> (273.8666, -10.7215)
  line L345 (273.8666, -10.7215) -> (273.8666, -11.5514)
  line L346 (271.2954, -11.5366) -> (269.5985, -11.5366)
  line L347 (269.5985, -11.5366) -> (269.0279, -13.8708)
  line L348 (269.0279, -13.8708) -> (270.7248, -13.8708)
  line L349 (270.7248, -13.8708) -> (271.2954, -11.5366)
  spline S74 degree 2 poles (292.505, -17.435) (291.6158, -17.435) (290.1115, -16.8348) (289.5632, -16.2346) knots 0 0 0 1 2 2 2
  spline S75 degree 2 poles (289.5632, -16.2346) (289.0148, -15.6418) (288.4146, -13.8634) (288.4146, -12.7074) knots 0 0 0 1 2 2 2
  spline S76 degree 2 poles (288.4146, -12.7074) (288.4146, -11.5589) (289, -9.8545) (289.5558, -9.2247) knots 0 0 0 1 2 2 2
  spline S77 degree 2 poles (289.5558, -9.2247) (290.1041, -8.6097) (291.6009, -7.965) (292.5272, -7.965) knots 0 0 0 1 2 2 2
  spline S78 degree 2 poles (292.5272, -7.965) (292.9866, -7.965) (293.7943, -8.0984) (294.1352, -8.2021) knots 0 0 0 1 2 2 2
  spline S79 degree 2 poles (294.1352, -8.2021) (294.4316, -8.2984) (295.0466, -8.5726) (295.3504, -8.7356) knots 0 0 0 1 2 2 2
  line L350 (295.3504, -8.7356) -> (295.3504, -10.2028)
  line L351 (295.3504, -10.2028) -> (295.2541, -10.2028)
  spline S80 degree 2 poles (295.2541, -10.2028) (295.0911, -10.0546) (294.5872, -9.6396) (294.2241, -9.4396) knots 0 0 0 1 2 2 2
  spline S81 degree 2 poles (294.2241, -9.4396) (293.8758, -9.2469) (293.0533, -9.0024) (292.5198, -9.0024) knots 0 0 0 1 2 2 2
  spline S82 degree 2 poles (292.5198, -9.0024) (291.9344, -9.0024) (290.8896, -9.484) (290.4969, -9.9435) knots 0 0 0 1 2 2 2
  spline S83 degree 2 poles (290.4969, -9.9435) (290.1115, -10.4103) (289.6817, -11.8256) (289.6817, -12.7074) knots 0 0 0 1 2 2 2
  spline S84 degree 2 poles (289.6817, -12.7074) (289.6817, -13.6485) (290.1338, -15.0045) (290.5265, -15.4714) knots 0 0 0 1 2 2 2
  spline S85 degree 2 poles (290.5265, -15.4714) (290.9118, -15.9234) (291.9418, -16.3828) (292.5198, -16.3828) knots 0 0 0 1 2 2 2
  spline S86 degree 2 poles (292.5198, -16.3828) (293.0459, -16.3828) (293.9425, -16.1234) (294.2908, -15.9308) knots 0 0 0 1 2 2 2
  spline S87 degree 2 poles (294.2908, -15.9308) (294.6242, -15.7381) (295.1207, -15.338) (295.2615, -15.1972) knots 0 0 0 1 2 2 2
  line L352 (295.2615, -15.1972) -> (295.3504, -15.1972)
  line L353 (295.3504, -15.1972) -> (295.3504, -16.6496)
  spline S88 degree 2 poles (295.3504, -16.6496) (295.0466, -16.7903) (294.5131, -17.0497) (294.1352, -17.1683) knots 0 0 0 1 2 2 2
  spline S89 degree 2 poles (294.1352, -17.1683) (293.735, -17.3016) (293.0533, -17.435) (292.505, -17.435) knots 0 0 0 1 2 2 2
  dimension "d26" = 304.8
  dimension "d27" = 25.4
  dimension "d28" = 19.05
  dimension "d29" = 3.175
  dimension "d30" = 1.27
  dimension "d31" = 24.765
  dimension "d32" = 24.765
  dimension "d33" = 12.7
  dimension "d34" = 12.7
  dimension "d35" = 6.35
  dimension "d36" = 6.0325
  dimension "d39" = 25.4
  dimension "d44" = 12.7
  dimension "d45" = 12.7
  dimension "d47" = 25.4
  dimension "d48" = 6.35
  dimension "d49" = 12.7
  dimension "d50" = 12.7
  dimension "d51" = 6.35
  dimension "d52" = 25.4
  dimension "d53" = 12.7
  dimension "d54" = 12.7
  dimension "d55" = 6.35
  dimension "d56" = 25.4
  dimension "d57" = 12.7
  dimension "d58" = 12.7
  dimension "d59" = 6.35
  dimension "d60" = 25.4
  dimension "d61" = 12.7
  dimension "d62" = 12.7
  dimension "d63" = 12.7
  dimension "d64" = 12.7
  dimension "d65" = 12.7
  dimension "d66" = 12.7
  dimension "d67" = 12.7
  dimension "d68" = 12.7
  dimension "d69" = 12.7
  dimension "d70" = 12.7
  dimension "d71" = 12.7
  dimension "d72" = 12.7
  dimension "d73" = 12.7
  dimension "d74" = 12.7
  dimension "d75" = 6.35
  dimension "d76" = 25.4
  dimension "d77" = 6.35
  dimension "d78" = 25.4
  dimension "d79" = 6.35
  dimension "d80" = 25.4
  dimension "d81" = 6.35
  dimension "d82" = 25.4
  dimension "d83" = 6.35
  dimension "d84" = 25.4
  dimension "d85" = 6.35
  dimension "d86" = 25.4
  dimension "d87" = 25.4
  dimension "d88" = 6.35
  constraints: 88 end point, 3 perpendicular, 1 horizontal, 1 vertical, 104 other
  measures "d26" distance of L0.start L0.end
  measures "d27" distance of L0.start L1.end
  measures "d28" distance of L4.start L4.end
  measures "d29" distance between parallel lines of L0 L7
  measures "d30" distance of L4.end L5.end
  measures "d31" distance between parallel lines of L1 L4
  measures "d32" distance from line of L1 L4.start
  measures "d33" distance of L10.end L8.start
  measures "d34" distance of L8.start L8.end
  measures "d35" distance between parallel lines of L0 L8
  measures "d36" distance between parallel lines of L1 L11
  measures "d39" distance of L4.end L12.end
  measures "d44" distance of L55.start L55.end
  measures "d45" distance of L55.end L52.end
  measures "d47" distance between parallel lines of L11 L55
  measures "d48" distance between parallel lines of L0 L52
  measures "d49" distance of L59.start L59.end
  measures "d50" distance of L59.end L56.end
  measures "d51" distance between parallel lines of L0 L56
  measures "d52" distance between parallel lines of L55 L59
  measures "d53" distance of L63.start L63.end
  measures "d54" distance of L63.end L60.end
  measures "d55" distance between parallel lines of L0 L60
  measures "d56" distance between parallel lines of L59 L63
  measures "d57" distance of L67.start L67.end
  measures "d58" distance of L67.end L64.end
  measures "d59" distance between parallel lines of L0 L64
  measures "d60" distance between parallel lines of L63 L67
  measures "d61" distance of L71.start L71.end
  measures "d62" distance of L71.end L68.end
  measures "d63" distance of L75.start L75.end
  measures "d64" distance of L75.end L72.end
  measures "d65" distance of L79.start L79.end
  measures "d66" distance of L79.end L76.end
  measures "d67" distance of L83.start L83.end
  measures "d68" distance of L83.end L80.end
  measures "d69" distance of L87.start L87.end
  measures "d70" distance of L87.end L84.end
  measures "d71" distance of L91.start L91.end
  measures "d72" distance of L91.end L88.end
  measures "d73" distance of L95.start L95.end
  measures "d74" distance of L95.end L92.end
  measures "d75" distance between parallel lines of L0 L68
  measures "d76" distance between parallel lines of L67 L71
  measures "d77" distance between parallel lines of L0 L72
  measures "d78" distance between parallel lines of L71 L75
  measures "d79" distance between parallel lines of L0 L76
  measures "d80" distance between parallel lines of L75 L79
  measures "d81" distance between parallel lines of L0 L80
  measures "d82" distance between parallel lines of L79 L83
  measures "d83" distance between parallel lines of L0 L84
  measures "d84" distance between parallel lines of L83 L87
  measures "d85" distance between parallel lines of L0 L88
  measures "d86" distance between parallel lines of L87 L91
  measures "d87" distance between parallel lines of L91 L95
  measures "d88" distance between parallel lines of L0 L92
extrude "Extrusion5" cut sketch "Sketch5" against normal blind 5.08 contours L7 L6 L5 L4 | L13 L15 L14 L12 | L17 L19 L18 L16 | L21 L23 L22 L20 | L25 L27 L26 L24 | L29 L31 L30 L28 | L33 L35 L34 L32 | L37 L39 L38 L36 | L41 L43 L42 L40 | L45 L47 L46 L44 | L49 L51 L50 L48 | L96 L97 L98 L99 L100 L101 L102 L103 | L107 L108 L109 L110 L111 L112 L113 L114 L115 L116 L117 L118 L119 L120 L121 L122 L123 L124 L125 L126 L127 L128 L129 L130 L131 L132 L133 L134 | S0 S1 L139 L140 L141 S2 S3 S4 L142 S5 | L149 L150 L151 L152 L153 L154 L155 L156 | S14 S15 S16 S17 S18 S19 L160 L161 S20 S21 S22 S23 S24 S25 L162 L163 L164 L165 L166 S26 S27 | L167 L168 L169 L170 L171 L172 L173 L174 L175 L176 L177 L178 L179 L180 L181 L182 L183 L184 L185 L186 L187 L188 L189 L190 L191 L192 L193 L194 | S28 S29 S30 S31 S32 S33 L199 L200 S34 S35 S36 S37 S38 S39 L201 L202 L203 L204 L205 S40 S41 | L206 L207 L208 L209 L210 L211 L212 L213 L214 L215 | L216 L217 L218 L219 L220 L221 L222 L223 L224 L225 L226 L227 L228 L229 L230 L231 L232 L233 L234 L235 L236 L237 L238 L239 L240 L241 L242 L243 | L248 L249 L250 L251 L252 L253 L254 L255 L256 L257 | L258 L259 L260 L261 L262 L263 L264 L265 L266 L267 L268 L269 | S42 S43 L270 L271 L272 S44 S45 | L276 L277 L278 L279 L280 L281 L282 L283 L284 L285 L286 L287 L288 L289 L290 L291 L292 L293 L294 L295 L296 L297 L298 L299 L300 L301 L302 L303 | S50 S51 L308 L309 L310 S52 S53 | S58 S59 S60 S61 S62 S63 L314 L315 S64 S65 S66 S67 S68 S69 S70 S71 L316 L317 S72 S73 | L318 L319 L320 L321 L322 L323 L324 L325 L326 L327 L328 L329 L330 L331 L332 L333 L334 L335 L336 L337 L338 L339 L340 L341 L342 L343 L344 L345 | S74 S75 S76 S77 S78 S79 L350 L351 S80 S81 S82 S83 S84 S85 S86 S87 L352 L353 S88 S89